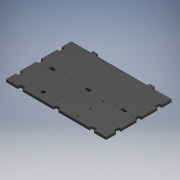
# Autodesk Inventor part: BA02
Saved by Autodesk Inventor 2017 (Build 210142000, 142)
## iProperties
Created: 2019-05-22
Part Number: BA02
Material: Wood (Cherry)
Document SubType Name: Modeling
Designer: Dell
Density: 0.63 g/cm^3
Appearance: Smooth - Black
Mass: 1410.59 g
Surface Area: 3861.69 cm^2
Volume: 2239.03 cm^3
Author: Dell
Autodesk Inventor part; units mm, degrees
ref_plane "YZ Plane" through (0, 0, 0) normal (1, 0, 0) x (0, 1, 0)
ref_plane "XZ Plane" through (0, 0, 0) normal (0, 1, 0) x (-1, 0, 0)
ref_plane "XY Plane" through (0, 0, 0) normal (0, 0, 1) x (1, 0, 0)
sketch "Sketch1" plane through (0, 0, 0) normal (0, 0, 1) x (1, 0, 0)
  line L0 (0, 0) -> (525.78, 0)
  line L1 (525.78, 0) -> (525.78, 342.9)
  line L2 (525.78, 342.9) -> (0, 342.9)
  line L3 (0, 342.9) -> (0, 0)
  line L4 (226.36, 66.95) -> (226.36, 21.95) construction
  circle A0 centre (226.36, 66.95) radius 2.3813
  circle A1 centre (226.36, 21.95) radius 2.3813
  circle A2 centre (226.36, 44.45) radius 2.3813
  line L5 (166.36, 29.45) -> (166.36, 49.45) construction
  line L6 (156.36, 66.95) -> (156.36, 21.95) construction
  line L7 (166.36, 49.45) -> (146.36, 49.45) construction
  line L8 (146.36, 29.45) -> (166.36, 29.45) construction
  circle A3 centre (156.36, 39.45) radius 10
  line L9 (226.36, 21.95) -> (86.36, 21.95) construction
  line L10 (86.36, 66.95) -> (226.36, 66.95) construction
  line L11 (86.36, 44.45) -> (226.36, 44.45) construction
  line L12 (146.36, 49.45) -> (146.36, 29.45) construction
  line L13 (0, 0) -> (525.78, 0) construction
  line L14 (525.78, 0) -> (525.78, 88.9)
  line L15 (525.78, 88.9) -> (0, 88.9) construction
  line L16 (0, 88.9) -> (0, 0) construction
  line L17 (86.36, 21.95) -> (86.36, 66.95) construction
  circle A4 centre (86.36, 66.95) radius 2.3812
  circle A5 centre (86.36, 21.95) radius 2.3812
  circle A6 centre (86.36, 44.45) radius 2.3812
  point P0 (166.36, 39.45)
  point P1 (146.36, 39.45)
  point P2 (0, 44.45)
  dimension "d0" = 342.9
  dimension "d1" = 525.78
  dimension "d2" = 45
  dimension "d3" = 140
  dimension "d4" = 4.7625
  dimension "d5" = 4.7625
  dimension "d6" = 4.7625
  dimension "d7" = 4.7625
  dimension "d8" = 4.7625
  dimension "d9" = 4.7625
  dimension "d10" = 60
  dimension "d11" = 7.5
  dimension "d12" = 20
  dimension "d13" = 20
  dimension "d14" = 86.36
  dimension "d15" = 88.9
  constraints: 36 end point, 8 parallel, 7 midpoint, 6 centre point, 5 coincident, 4 perpendicular, 3 horizontal alignment, 2 horizontal, 2 point on line, 2 other
  measures "d0" distance of L2.end L0.start
  measures "d1" distance of L0.start L0.end
  measures "d2" distance of L4.start L4.end
  measures "d3" distance of L17.end L4.start
  measures "d4" diameter of A4
  measures "d5" diameter of A6
  measures "d6" diameter of A5
  measures "d7" diameter of A1
  measures "d8" diameter of A2
  measures "d9" diameter of A0
  measures "d10" distance from line of L11.end L5
  measures "d11" distance between parallel lines of L9 L8
  measures "d12" distance of L5.end L12.start
  measures "d13" distance of L12.start L8.start
  measures "d14" distance between parallel lines of L16 L17
  measures "d15" distance of L15.end L13.start
extrude "Extrusion1" add sketch "Sketch1" along normal blind 12.7
sketch "Sketch2" plane through (0, 0, 12.7) normal (0, 0, 1) x (1, 0, 0)
  line L0 (525.78, 342.9) -> (0, 342.9) projected
  line L1 (101.6, 342.9) -> (127, 342.9)
  line L2 (127, 342.9) -> (127, 355.6)
  line L3 (127, 355.6) -> (101.6, 355.6)
  line L4 (101.6, 355.6) -> (101.6, 342.9)
  line L5 (0, 342.9) -> (0, 0) projected
  line L6 (262.89, 342.9) -> (262.89, 386.8153)
  line L7 (0, 342.9) -> (525.78, 342.9)
  line L8 (424.18, 342.9) -> (398.78, 342.9)
  line L9 (398.78, 342.9) -> (398.78, 355.6)
  line L10 (398.78, 355.6) -> (424.18, 355.6)
  line L11 (424.18, 355.6) -> (424.18, 342.9)
  dimension "d18" = 25.4
  dimension "d19" = 12.7
  dimension "d20" = 101.6
  constraints: 20 end point, 6 symmetric about line, 2 parallel, 2 point on line, 1 horizontal, 1 midpoint, 1 perpendicular, 1 vertical
  measures "d18" distance of L3.end L2.end
  measures "d19" distance of L2.end L1.end
  measures "d20" distance from line of L5 L3.end
extrude "Extrusion2" add sketch "Sketch2" against normal blind 12.7
sketch "Sketch3" plane through (0, 0, 12.7) normal (0, 0, 1) x (1, 0, 0)
  line L0 (101.6, 355.6) -> (101.6, 342.9) projected
  line L1 (127, 355.6) -> (101.6, 355.6) projected
  line L2 (424.18, 355.6) -> (424.18, 342.9) projected
  line L3 (398.78, 355.6) -> (424.18, 355.6) projected
  circle A0 centre (114.3, 349.25) radius 2.25
  circle A1 centre (411.48, 349.25) radius 2.25
  point P0 (0, 0)
  point P1 (114.3, 355.6)
  point P2 (101.6, 349.25)
  point P3 (424.18, 349.25)
  point P4 (411.48, 355.6)
  dimension "d23" = 4.5
  dimension "d24" = 4.5
  constraints: 4 midpoint, 2 centre point, 2 horizontal alignment, 2 vertical alignment
  measures "d23" diameter of A0
  measures "d24" diameter of A1
extrude "Extrusion3" cut sketch "Sketch3" against normal through all
sketch "Sketch4" plane through (0, 0, 12.7) normal (0, 0, 1) x (1, 0, 0)
  line L0 (0, 342.9) -> (0, 0) projected
  line L1 (0, 292.1) -> (12.7, 292.1)
  line L2 (12.7, 292.1) -> (12.7, 266.7)
  line L3 (12.7, 266.7) -> (0, 266.7)
  line L4 (0, 266.7) -> (0, 292.1)
  line L5 (0, 184.15) -> (12.7, 184.15)
  line L6 (12.7, 184.15) -> (12.7, 158.75)
  line L7 (12.7, 158.75) -> (0, 158.75)
  line L8 (0, 158.75) -> (0, 184.15)
  line L9 (0, 50.8) -> (12.7, 50.8)
  line L10 (12.7, 50.8) -> (12.7, 76.2)
  line L11 (12.7, 76.2) -> (0, 76.2)
  line L12 (0, 76.2) -> (0, 50.8)
  line L13 (398.78, 342.9) -> (127, 342.9) projected
  line L14 (262.89, 342.9) -> (262.89, 381.8004)
  line L15 (525.78, 342.9) -> (525.78, 0)
  line L16 (525.78, 292.1) -> (513.08, 292.1)
  line L17 (513.08, 292.1) -> (513.08, 266.7)
  line L18 (513.08, 266.7) -> (525.78, 266.7)
  line L19 (525.78, 266.7) -> (525.78, 292.1)
  line L20 (525.78, 184.15) -> (513.08, 184.15)
  line L21 (513.08, 184.15) -> (513.08, 158.75)
  line L22 (513.08, 158.75) -> (525.78, 158.75)
  line L23 (525.78, 158.75) -> (525.78, 184.15)
  line L24 (525.78, 50.8) -> (513.08, 50.8)
  line L25 (513.08, 50.8) -> (513.08, 76.2)
  line L26 (513.08, 76.2) -> (525.78, 76.2)
  line L27 (525.78, 76.2) -> (525.78, 50.8)
  point P0 (0, 171.45)
  point P1 (525.78, 171.45)
  dimension "d27" = 12.7
  dimension "d28" = 25.4
  dimension "d29" = 12.7
  dimension "d30" = 25.4
  dimension "d31" = 12.7
  dimension "d32" = 25.4
  dimension "d33" = 50.8
  dimension "d34" = 50.8
  constraints: 52 end point, 15 symmetric about line, 6 parallel, 6 point on line, 3 horizontal, 3 midpoint, 3 perpendicular, 1 vertical
  measures "d27" distance of L2.end L3.end
  measures "d28" distance of L1.end L2.end
  measures "d29" distance of L6.end L7.end
  measures "d30" distance of L5.end L6.end
  measures "d31" distance of L11.end L10.end
  measures "d32" distance of L9.end L10.end
  measures "d33" distance from line of L0.start L1
  measures "d34" distance from line of L0.end L9
extrude "Extrusion4" cut sketch "Sketch4" against normal through all
sketch "Sketch5" plane through (0, 0, 0) normal (0, -1, 0) x (1, 0, 0)
  line L0 (62.69, 12.7) -> (88.09, 12.7)
  line L1 (88.09, 12.7) -> (88.09, 0)
  line L2 (88.09, 0) -> (62.69, 0)
  line L3 (62.69, 0) -> (62.69, 12.7)
  line L4 (250.19, 12.7) -> (275.59, 12.7)
  line L5 (275.59, 12.7) -> (275.59, 0)
  line L6 (275.59, 0) -> (250.19, 0)
  line L7 (250.19, 0) -> (250.19, 12.7)
  line L8 (437.69, 12.7) -> (463.09, 12.7)
  line L9 (463.09, 12.7) -> (463.09, 0)
  line L10 (463.09, 0) -> (437.69, 0)
  line L11 (437.69, 0) -> (437.69, 12.7)
  line L12 (75.39, 0) -> (450.39, 0) construction
  line L13 (0, 0) -> (525.78, 0) projected
  point P0 (262.89, 12.7)
  point P1 (262.89, 12.7)
  point P2 (262.89, 0)
  dimension "d37" = 25.4
  dimension "d38" = 12.7
  dimension "d39" = 25.4
  dimension "d40" = 12.7
  dimension "d41" = 25.4
  dimension "d42" = 12.7
  dimension "d43" = 375
  constraints: 26 end point, 6 midpoint, 6 parallel, 3 horizontal, 3 perpendicular, 1 point on line, 1 vertical alignment
  measures "d37" distance of L1.end L2.end
  measures "d38" distance of L1.start L1.end
  measures "d39" distance of L6.start L7.start
  measures "d40" distance of L4.end L6.start
  measures "d41" distance of L9.end L10.end
  measures "d42" distance of L8.end L9.end
  measures "d43" distance of L12.start L12.end
extrude "Extrusion5" cut sketch "Sketch5" against normal blind 12.7
sketch "Sketch6" plane through (0, 0, 12.7) normal (0, 0, 1) x (1, 0, 0)
  line L0 (62.69, 174.15) -> (88.09, 174.15)
  line L1 (88.09, 174.15) -> (88.09, 161.45)
  line L2 (88.09, 161.45) -> (62.69, 161.45)
  line L3 (62.69, 161.45) -> (62.69, 174.15)
  line L4 (250.19, 161.45) -> (275.59, 161.45)
  line L5 (275.59, 161.45) -> (275.59, 174.15)
  line L6 (275.59, 174.15) -> (250.19, 174.15)
  line L7 (250.19, 174.15) -> (250.19, 161.45)
  line L8 (437.69, 161.45) -> (463.09, 161.45)
  line L9 (463.09, 161.45) -> (463.09, 174.15)
  line L10 (463.09, 174.15) -> (437.69, 174.15)
  line L11 (437.69, 174.15) -> (437.69, 161.45)
  line L12 (12.7, 184.15) -> (12.7, 158.75) projected
  line L13 (62.69, 12.7) -> (88.09, 12.7) projected
  line L14 (250.19, 12.7) -> (275.59, 12.7) projected
  line L15 (437.69, 12.7) -> (463.09, 12.7) projected
  point P0 (0, 0)
  dimension "d48" = 12.7
  dimension "d49" = 10
  constraints: 24 end point, 6 parallel, 6 vertical alignment, 3 horizontal, 3 horizontal alignment, 3 perpendicular, 1 point on line
  measures "d48" distance of L0.end L1.end
  measures "d49" distance from line of L12.start L0
extrude "Extrusion6" cut sketch "Sketch6" against normal through all
sketch "Sketch7" plane through (0, 0, 12.7) normal (0, 0, 1) x (1, 0, 0)
  line L0 (275.59, 0) -> (437.69, 0) construction
  line L1 (331.24, 0) -> (382.04, 0) construction
  line L2 (382.04, 0) -> (382.04, 174.15) construction
  line L3 (382.04, 174.15) -> (331.24, 174.15) construction
  line L4 (331.24, 174.15) -> (331.24, 0) construction
  circle A0 centre (356.64, 154.15) radius 4
  circle A1 centre (356.64, 87.075) radius 4
  circle A2 centre (356.64, 20) radius 4
  circle A3 centre (305.84, 167.8) radius 2.25
  circle A4 centre (407.44, 167.8) radius 2.25
  circle A5 centre (305.84, 6.35) radius 2.25
  circle A6 centre (407.44, 6.35) radius 2.25
  line L5 (275.59, 12.7) -> (275.59, 0) projected
  line L6 (437.69, 161.45) -> (437.69, 174.15) projected
  point P0 (0, 0)
  point P1 (275.59, 174.15)
  point P2 (356.64, 0)
  point P3 (356.64, 174.15)
  point P4 (382.04, 87.075)
  point P5 (275.59, 6.35)
  point P6 (437.69, 167.8)
  dimension "d50" = 50.8
  dimension "d51" = 8
  dimension "d52" = 8
  dimension "d53" = 8
  dimension "d54" = 20
  dimension "d55" = 20
  dimension "d72" = 4.5
  dimension "d73" = 4.5
  dimension "d74" = 4.5
  dimension "d75" = 4.5
  dimension "d76" = 25.4
  dimension "d77" = 25.4
  constraints: 8 end point, 7 centre point, 6 horizontal alignment, 6 midpoint, 5 vertical alignment, 2 parallel, 1 horizontal, 1 perpendicular, 1 point on line
  measures "d50" distance of L3.end L2.end
  measures "d51" diameter of A0
  measures "d52" diameter of A1
  measures "d53" diameter of A2
  measures "d54" distance from line of L3 A0.centre
  measures "d55" distance from line of L0 A2.centre
  measures "d72" diameter of A3
  measures "d73" diameter of A4
  measures "d74" diameter of A5
  measures "d75" diameter of A6
  measures "d76" distance from line of A3.centre L4
  measures "d77" distance from line of A4.centre L2
extrude "Extrusion7" cut sketch "Sketch7" against normal through all
sketch "Sketch8" plane through (0, 0, 12.7) normal (0, 0, 1) x (1, 0, 0)
  line L0 (62.69, 161.45) -> (62.69, 174.15) projected
  line L1 (12.7, 184.15) -> (12.7, 158.75) projected
  line L2 (88.09, 174.15) -> (88.09, 161.45) projected
  line L3 (250.19, 161.45) -> (250.19, 174.15) projected
  line L4 (275.59, 174.15) -> (275.59, 161.45) projected
  line L5 (463.09, 174.15) -> (463.09, 161.45) projected
  line L6 (513.08, 158.75) -> (513.08, 184.15) projected
  line L7 (62.69, 0) -> (62.69, 12.7) projected
  line L8 (250.19, 0) -> (250.19, 12.7) projected
  line L9 (275.59, 12.7) -> (275.59, 0) projected
  line L10 (437.69, 0) -> (437.69, 12.7) projected
  line L11 (463.09, 12.7) -> (463.09, 0) projected
  circle A0 centre (31.345, 6.35) radius 2.25
  circle A1 centre (169.14, 6.35) radius 2.25
  circle A2 centre (494.435, 6.35) radius 2.25
  circle A3 centre (494.435, 167.8) radius 2.25
  circle A4 centre (169.14, 167.8) radius 2.25
  circle A5 centre (31.345, 167.8) radius 2.25
  line L12 (88.09, 0) -> (250.19, 0) projected
  line L13 (0, 0) -> (62.69, 0) projected
  line L14 (463.09, 0) -> (525.78, 0) projected
  point P0 (62.69, 6.35)
  point P1 (62.69, 6.35)
  point P2 (275.59, 6.35)
  point P3 (463.09, 6.35)
  point P4 (463.09, 167.8)
  point P5 (250.19, 167.8)
  point P6 (62.69, 167.8)
  point P7 (169.14, 0)
  point P8 (31.345, 0)
  point P9 (494.435, 0)
  dimension "d58" = 4.5
  dimension "d59" = 4.5
  dimension "d60" = 4.5
  dimension "d61" = 4.5
  dimension "d62" = 4.5
  dimension "d63" = 4.5
  constraints: 10 midpoint, 6 centre point, 6 horizontal alignment, 6 vertical alignment
  measures "d58" diameter of A0
  measures "d59" diameter of A1
  measures "d60" diameter of A2
  measures "d61" diameter of A3
  measures "d62" diameter of A4
  measures "d63" diameter of A5
extrude "Extrusion8" cut sketch "Sketch8" against normal through all
equation "\"d40\" = d38"
equation "\"d42\" = d40"
body "Solid1"
